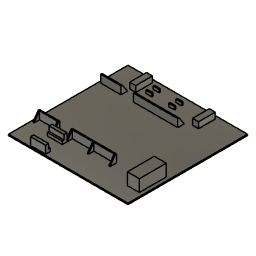
dysk v3 (Autodesk Fusion 360 design; units mm, degrees)
Autodesk Fusion 360 part; units mm, degrees
note: some values were not read from the file. Chosen so that the rebuilt part matches the saved one: which bodies a step acts on.
sketch "Szkic1" plane through (0, 0, 0) normal (0, 0, 1) x (1, 0, 0)
  line L0 (-100, 100) -> (100, 100)
  line L1 (100, 100) -> (100, -100)
  line L2 (100, -100) -> (-100, -100)
  line L3 (-100, -100) -> (-100, 100)
  dimension "d1" = 200
  dimension "d2" = 200
  constraint horizontal L0
  constraint vertical L1
  constraint horizontal L2
  constraint vertical L3
  measures "d1" distance of L0.start L0.end
  measures "d2" distance of L0.start L2.end
extrude "Wyciągnięcie proste1" add sketch "Szkic1" along normal blind 2 makes body 1
sketch "Szkic2" plane through (0, 0, 2) normal (0, 0, 1) x (-1, 0, 0)
  line L0 (100, 100) -> (-100, 100)
  line L1 (-100, 100) -> (-100, -100)
  line L2 (-100, -100) -> (100, -100)
  line L3 (100, -100) -> (100, 100)
  line L4 (95, 51) -> (65, 51)
  line L5 (95, 51) -> (65, 51)
  line L6 (65, 51) -> (65, 53)
  line L7 (65, 53) -> (95, 53)
  line L8 (95, 53) -> (95, 51)
  line L9 (95, -51) -> (65, -51)
  line L10 (65, -51) -> (65, -53)
  line L11 (65, -53) -> (95, -53)
  line L12 (95, -53) -> (95, -51)
  line L13 (40, -53) -> (-30, -53)
  line L14 (-30, -53) -> (-30, -51)
  line L15 (-30, -51) -> (40, -51)
  line L16 (40, -51) -> (40, -53)
  line L17 (40, 51) -> (-30, 51)
  line L18 (-30, 51) -> (-30, 53)
  line L19 (-30, 53) -> (40, 53)
  line L20 (40, 53) -> (40, 51)
  dimension "d10" = 30
  dimension "d11" = 5
  constraint horizontal L4
  constraint horizontal L5
  constraint vertical L6
  constraint horizontal L7
  constraint vertical L8
  constraint horizontal L9
  constraint vertical L10
  constraint horizontal L11
  constraint vertical L12
  constraint horizontal L13
  constraint vertical L14
  constraint horizontal L15
  constraint vertical L16
  constraint horizontal L17
  constraint vertical L18
  constraint horizontal L19
  constraint vertical L20
  measures "d10" distance of L10.end L11.end
  measures "d11" distance of L3 L12
extrude "Wyciągnięcie proste2" add sketch "Szkic2" along normal blind 13 separate body contours L4 L5 L6 L7 L8 | L9 L10 L11 L12 | L13 L14 L15 L16 | L17 L18 L19 L20 makes body 2 at (-16.6667, 53, 6.3333) makes body 3 at (-75, -53, 6.3333) makes body 4 at (-16.6667, -51, 6.3333) makes body 5 at (-75, 53, 6.3333)
sketch "Szkic3" plane through (-95, 0, 0) normal (-1, 0, 0) x (0, -1, 0)
  line L0 (51, 2) -> (53, 2)
  line L1 (53, 2) -> (53, 15)
  line L2 (53, 15) -> (51, 15)
  line L3 (51, 15) -> (51, 2)
  line L4 (53, 15) -> (62, 2)
  line L5 (62, 2) -> (51, 2)
  constraint coincident L1.end L2.start
  constraint coincident L0.start L3.end
extrude "Wyciągnięcie proste3" add sketch "Szkic3" along normal blind 2 separate body makes body 6
sketch "Szkic4" plane through (-95, 0, 0) normal (-1, 0, 0) x (0, -1, 0)
  line L0 (-53, 2) -> (-51, 2)
  line L1 (-51, 2) -> (-51, 15)
  line L2 (-51, 15) -> (-53, 15)
  line L3 (-53, 15) -> (-53, 2)
  line L4 (-53, 15) -> (-62, 2)
  line L5 (-62, 2) -> (-51, 2)
  constraint coincident L2.end L3.start
  constraint coincident L0.end L1.start
extrude "Wyciągnięcie proste4" add sketch "Szkic4" along normal blind 2 bodies 1 5
sketch "Szkic5" plane through (-65, 0, 0) normal (1, 0, 0) x (0, 1, 0)
  line L0 (51, 2) -> (53, 2)
  line L1 (53, 2) -> (53, 15)
  line L2 (53, 15) -> (51, 15)
  line L3 (51, 15) -> (51, 2)
  line L4 (53, 15) -> (62, 2)
  line L5 (62, 2) -> (51, 2)
  constraint coincident L1.end L2.start
  constraint coincident L0.start L3.end
extrude "Wyciągnięcie proste5" add sketch "Szkic5" along normal blind 2 bodies 1
sketch "Szkic6" plane through (-65, 0, 0) normal (1, 0, 0) x (0, 1, 0)
  line L0 (-53, 2) -> (-51, 2)
  line L1 (-51, 2) -> (-51, 15)
  line L2 (-51, 15) -> (-53, 15)
  line L3 (-53, 15) -> (-53, 2)
  line L4 (-53, 15) -> (-62, 2)
  line L5 (-62, 2) -> (-51, 2)
  constraint coincident L2.end L3.start
  constraint coincident L0.end L1.start
extrude "Wyciągnięcie proste6" add 1 faces at (30, -51.6667, 6.3333) along direction (1, 0, 0) blind 2 on bodies 4 bodies 1 2 3 6 4
extrude "Wyciągnięcie proste7" add sketch "Szkic6" along normal blind 2 bodies 1 6 3
sketch "Szkic7" plane through (-40, 0, 0) normal (-1, 0, 0) x (0, -1, 0)
  line L0 (51, 2) -> (53, 2)
  line L1 (53, 2) -> (53, 15)
  line L2 (53, 15) -> (51, 15)
  line L3 (51, 15) -> (51, 2)
  line L4 (53, 15) -> (62, 2)
  line L5 (62, 2) -> (51, 2)
  constraint coincident L1.end L2.start
  constraint coincident L0.start L3.end
extrude "Wyciągnięcie proste8" add sketch "Szkic7" along normal blind 2 bodies 1
sketch "Szkic8" plane through (32, 0, 0) normal (1, 0, 0) x (0, 1, 0)
  line L0 (-53, 2) -> (-51, 2)
  line L1 (-51, 2) -> (-51, 15)
  line L2 (-51, 15) -> (-53, 15)
  line L3 (-53, 15) -> (-53, 2)
  line L4 (-53, 15) -> (-62, 2)
  line L5 (-62, 2) -> (-51, 2)
  constraint coincident L2.end L3.start
  constraint coincident L0.end L1.start
extrude "Wyciągnięcie proste9" add sketch "Szkic8" along normal blind 2 bodies 1
sketch "Szkic9" plane through (30, 0, 0) normal (1, 0, 0) x (0, 1, 0)
  line L0 (51, 2) -> (53, 2)
  line L1 (53, 2) -> (53, 15)
  line L2 (53, 15) -> (51, 15)
  line L3 (51, 15) -> (51, 2)
  line L4 (53, 15) -> (62, 2)
  line L5 (62, 2) -> (51, 2)
  constraint coincident L1.end L2.start
  constraint coincident L0.start L3.end
extrude "Wyciągnięcie proste10" add sketch "Szkic9" along normal blind 2 bodies 1 2
sketch "Szkic10" plane through (-40, 0, 0) normal (-1, 0, 0) x (0, -1, 0)
  line L0 (-53, 2) -> (-51, 2)
  line L1 (-51, 2) -> (-51, 15)
  line L2 (-51, 15) -> (-53, 15)
  line L3 (-53, 15) -> (-53, 2)
  line L4 (-53, 15) -> (-62, 2)
  line L5 (-62, 2) -> (-51, 2)
  constraint coincident L2.end L3.start
  constraint coincident L0.end L1.start
extrude "Wyciągnięcie proste11" add sketch "Szkic10" along normal blind 2 bodies 1
sketch "Szkic11" plane through (0, 0, 2) normal (0, 0, 1) x (-1, 0, 0)
  line L0 (40, -62) -> (40, -53)
  line L1 (40, -53) -> (-30, -53)
  line L2 (-30, -53) -> (-30, -62)
  line L3 (-30, -62) -> (-32, -62)
  line L4 (-32, -62) -> (-32, -51)
  line L5 (-32, -51) -> (42, -51)
  line L6 (42, -51) -> (42, -62)
  line L7 (42, -62) -> (40, -62)
  line L8 (63, -51) -> (97, -51)
  line L9 (97, -51) -> (97, -62)
  line L10 (97, -62) -> (95, -62)
  line L11 (95, -62) -> (95, -53)
  line L12 (95, -53) -> (65, -53)
  line L13 (65, -53) -> (65, -62)
  line L14 (65, -62) -> (63, -62)
  line L15 (63, -62) -> (63, -51)
  line L16 (100, 100) -> (-100, 100)
  line L17 (-100, 100) -> (-100, -100)
  line L18 (-100, -100) -> (100, -100)
  line L19 (100, -100) -> (100, 100)
  line L20 (65, 62) -> (65, 53)
  line L21 (65, 53) -> (95, 53)
  line L22 (95, 53) -> (95, 51)
  line L23 (95, 51) -> (63, 51)
  line L24 (63, 51) -> (63, 62)
  line L25 (63, 62) -> (65, 62)
  line L26 (42, 51) -> (-34, 51)
  line L27 (-34, 51) -> (-34, 62)
  line L28 (-34, 62) -> (-32, 62)
  line L29 (-32, 62) -> (-32, 53)
  line L30 (-32, 53) -> (40, 53)
  line L31 (40, 53) -> (40, 62)
  line L32 (40, 62) -> (42, 62)
  line L33 (42, 62) -> (42, 51)
  line L34 (4, -53) -> (6, -53)
  line L35 (6, -53) -> (6, -62)
  line L36 (6, -62) -> (4, -62)
  line L37 (4, -62) -> (4, -53)
  dimension "d32" = 34
  dimension "d33" = 2
  constraint horizontal L34
  constraint vertical L35
  constraint horizontal L36
  constraint vertical L37
  constraint coincident L1 L34.start
  measures "d32" distance of L2 L37
  measures "d33" distance of L35.end L36.end
sketch "Szkic12" plane through (-6, 0, 0) normal (-1, 0, 0) x (0, -1, 0)
  line L0 (-62, 2) -> (-53, 2)
  line L1 (-53, 2) -> (-53, 15)
  line L2 (-53, 15) -> (-62, 15)
  line L3 (-62, 15) -> (-62, 2)
  line L4 (-53, 15) -> (-62, 2)
  line L5 (-53, 15) -> (-62, 2)
  line L6 (-51, 2) -> (-51, 15)
  line L7 (-51, 15) -> (-53, 15)
  constraint coincident L1.end L2.start
  constraint coincident L0.start L3.end
  constraint perpendicular L0 L6
  constraint perpendicular L1 L7
extrude "Wyciągnięcie proste13" add sketch "Szkic12" against normal blind 2 contours L0 L1 L4 L5 bodies 1
sketch "Szkic13" plane through (0, 0, 2) normal (0, 0, 1) x (-1, 0, 0)
  line L0 (4, -62) -> (4, -53)
  line L1 (4, -53) -> (-30, -53)
  line L2 (-30, -53) -> (-30, -62)
  line L3 (-30, -62) -> (-32, -62)
  line L4 (-32, -62) -> (-32, -51)
  line L5 (-32, -51) -> (42, -51)
  line L6 (42, -51) -> (42, -62)
  line L7 (42, -62) -> (40, -62)
  line L8 (40, -62) -> (40, -53)
  line L9 (40, -53) -> (6, -53)
  line L10 (6, -53) -> (6, -62)
  line L11 (6, -62) -> (4, -62)
  line L12 (63, -51) -> (97, -51)
  line L13 (97, -51) -> (97, -62)
  line L14 (97, -62) -> (95, -62)
  line L15 (95, -62) -> (95, -53)
  line L16 (95, -53) -> (65, -53)
  line L17 (65, -53) -> (65, -62)
  line L18 (65, -62) -> (63, -62)
  line L19 (63, -62) -> (63, -51)
  line L20 (100, 100) -> (-100, 100)
  line L21 (-100, 100) -> (-100, -100)
  line L22 (-100, -100) -> (100, -100)
  line L23 (100, -100) -> (100, 100)
  line L24 (65, 62) -> (65, 53)
  line L25 (65, 53) -> (95, 53)
  line L26 (95, 53) -> (95, 51)
  line L27 (95, 51) -> (63, 51)
  line L28 (63, 51) -> (63, 62)
  line L29 (63, 62) -> (65, 62)
  line L30 (42, 51) -> (-34, 51)
  line L31 (-34, 51) -> (-34, 62)
  line L32 (-34, 62) -> (-32, 62)
  line L33 (-32, 62) -> (-32, 53)
  line L34 (-32, 53) -> (40, 53)
  line L35 (40, 53) -> (40, 62)
  line L36 (40, 62) -> (42, 62)
  line L37 (42, 62) -> (42, 51)
  line L38 (6, 53) -> (2, 53)
  line L39 (2, 53) -> (2, 61)
  line L40 (2, 61) -> (6, 61)
  line L41 (6, 61) -> (6, 53)
  dimension "d38" = 34
  dimension "d39" = 34
  constraint horizontal L38
  constraint vertical L39
  constraint horizontal L40
  constraint vertical L41
  constraint coincident L34 L38.start
  measures "d38" distance of L35 L41
  measures "d39" distance of L33 L39
extrude "Wyciągnięcie proste14" add 1 faces at (34, -56, 6.3333) along direction (-1, 0, 0) blind 4 on bodies 1 bodies 1
extrude "Wyciągnięcie proste15" cut 1 faces at (34, -56, 6.3333) along direction (-1, 0, 0) blind 2 on bodies 1 bodies 1
sketch "Szkic14" plane through (0, 0, 2) normal (0, 0, 1) x (-1, 0, 0)
  line L0 (-30, 62) -> (-30, 53)
  line L1 (-30, 53) -> (40, 53)
  line L2 (40, 53) -> (40, 62)
  line L3 (40, 62) -> (42, 62)
  line L4 (42, 62) -> (42, 51)
  line L5 (42, 51) -> (-32, 51)
  line L6 (-32, 51) -> (-32, 62)
  line L7 (-32, 62) -> (-30, 62)
  line L8 (4, -62) -> (4, -53)
  line L9 (4, -53) -> (-30, -53)
  line L10 (-30, -53) -> (-30, -62)
  line L11 (-30, -62) -> (-32, -62)
  line L12 (-32, -62) -> (-32, -51)
  line L13 (-32, -51) -> (42, -51)
  line L14 (42, -51) -> (42, -62)
  line L15 (42, -62) -> (40, -62)
  line L16 (40, -62) -> (40, -53)
  line L17 (40, -53) -> (6, -53)
  line L18 (6, -53) -> (6, -62)
  line L19 (6, -62) -> (4, -62)
  line L20 (63, -51) -> (97, -51)
  line L21 (97, -51) -> (97, -62)
  line L22 (97, -62) -> (95, -62)
  line L23 (95, -62) -> (95, -53)
  line L24 (95, -53) -> (65, -53)
  line L25 (65, -53) -> (65, -62)
  line L26 (65, -62) -> (63, -62)
  line L27 (63, -62) -> (63, -51)
  line L28 (100, 100) -> (-100, 100)
  line L29 (-100, 100) -> (-100, -100)
  line L30 (-100, -100) -> (100, -100)
  line L31 (100, -100) -> (100, 100)
  line L32 (65, 62) -> (65, 53)
  line L33 (65, 53) -> (95, 53)
  line L34 (95, 53) -> (95, 51)
  line L35 (95, 51) -> (63, 51)
  line L36 (63, 51) -> (63, 62)
  line L37 (63, 62) -> (65, 62)
sketch "Szkic15" plane through (0, 0, 2) normal (0, 0, 1) x (-1, 0, 0)
  line L0 (6, 62) -> (4, 62)
  line L1 (4, 62) -> (4, 53)
  line L2 (4, 53) -> (6, 53)
  line L3 (6, 53) -> (6, 62)
  line L4 (-30, 53) -> (40, 53)
  line L5 (40, 53) -> (40, 62)
  dimension "d44" = 34
  dimension "d45" = 9
  constraint horizontal L0
  constraint vertical L1
  constraint horizontal L2
  constraint vertical L3
  constraint coincident L1.end L4
  measures "d44" distance of L3 L5
  measures "d45" distance of L0.start L2.end
sketch "Szkic16" plane through (-4, 0, 0) normal (1, 0, 0) x (0, 1, 0)
  line L0 (-62, 2) -> (-53, 2)
  line L1 (-53, 2) -> (-53, 15)
  line L2 (-53, 15) -> (-62, 15)
  line L3 (-62, 15) -> (-62, 2)
  line L4 (-53, 15) -> (-62, 2)
  line L5 (-51, 2) -> (-51, 15)
  line L6 (-51, 15) -> (-53, 15)
  constraint coincident L1.end L2.start
  constraint coincident L0.start L3.end
  constraint perpendicular L0 L5
  constraint perpendicular L1 L6
extrude "Wyciągnięcie proste17" add sketch "Szkic16" against normal blind 2 contours L0 L1 L4 bodies 1
sketch "Szkic17" plane through (0, 0, 2) normal (0, 0, 1) x (-1, 0, 0)
sketch "Sketch18" plane through (0, 0, 2) normal (0, 0, 1) x (-1, 0, 0)
split "Split1" by plane through (0, 0, 2) normal (0, 0, 1) bodies 1 makes body 7 at (7.3333, -51, 6.3333) makes body 8 at (-85.6667, 51, 10.6667) makes body 9 at (-84.3333, -51, 6.3333) makes body 10 at (-17.3333, 51, 6.3333)
combine "Combine1" operation add target body 6 tool bodies 9
move_body "Move1" bodies 6 7 to x (1, 0, 0) y (0, 1, 0) z (0, 0, 1) at (0, -0.2, 0)
move_body "Move2" bodies 8 10 to x (1, 0, 0) y (0, 1, 0) z (0, 0, 1) at (0, 0.2, 0)
sketch "Sketch19" plane through (0, 0, 2) normal (0, 0, 1) x (-1, 0, 0)
  line L0 (100, 100) -> (-100, 100)
  line L1 (-100, 100) -> (-100, -100)
  line L2 (-100, -100) -> (100, -100)
  line L3 (100, -100) -> (100, 100)
  line L4 (-3.9507, -74.0001) -> (6, -74.0001)
  line L5 (6, -74.0001) -> (6, -76)
  line L6 (6, -76) -> (-3.9507, -76)
  line L7 (-3.9507, -76) -> (-3.9507, -74.0001)
  line L8 (-4, -86) -> (6, -86)
  line L9 (6, -86) -> (6, -88)
  line L10 (6, -88) -> (-4, -88)
  line L11 (-4, -88) -> (-4, -86)
  line L12 (34, -73.992) -> (44.0493, -73.992)
  line L13 (44.0493, -73.992) -> (44.0493, -76)
  line L14 (44.0493, -76) -> (34, -76)
  line L15 (34, -76) -> (34, -73.992)
  line L16 (34, -86) -> (44, -86)
  line L17 (44, -86) -> (44, -88)
  line L18 (44, -88) -> (34, -88)
  line L19 (34, -88) -> (34, -86)
  line L20 (54, -67) -> (64, -67)
  line L21 (64, -67) -> (64, -95)
  line L22 (64, -95) -> (54, -95)
  line L23 (54, -95) -> (54, -67)
  line L24 (-28, -67) -> (-38, -67)
  line L25 (-38, -67) -> (-38, -95)
  line L26 (-38, -95) -> (-28, -95)
  line L27 (-28, -95) -> (-28, -67)
  dimension "d50" = 14
  dimension "d51" = 48
  dimension "d52" = 48
  dimension "d56" = 10
  dimension "d57" = 28
  constraint horizontal L4
  constraint vertical L5
  constraint horizontal L6
  constraint vertical L7
  constraint horizontal L8
  constraint vertical L9
  constraint horizontal L10
  constraint vertical L11
  constraint horizontal L12
  constraint vertical L13
  constraint horizontal L14
  constraint vertical L15
  constraint horizontal L16
  constraint vertical L17
  constraint horizontal L18
  constraint vertical L19
  constraint horizontal L20
  constraint vertical L21
  constraint horizontal L22
  constraint vertical L23
  constraint horizontal L24
  constraint vertical L25
  constraint horizontal L26
  constraint vertical L27
  measures "d50" distance of L4.start L10.end
  measures "d51" distance of L4.start L12.end
  measures "d52" distance of L10.end L17.end
  measures "d56" distance of L20.start L20.end
  measures "d57" distance of L20.start L22.end
extrude "Extrude18" add sketch "Sketch19" along normal blind 5 separate body contours L4 L5 L6 L7 | L8 L9 L10 L11 | L12 L13 L14 L15 | L16 L17 L18 L19 makes body 11 at (-37.3498, 73.992, 5.3333) makes body 12 at (-37.3333, 86, 3.6667) makes body 13 at (0.6338, 74.0001, 3.6667) makes body 14 at (0.6667, 86, 3.6667)
extrude "Extrude19" add sketch "Sketch19" along normal blind 10 separate body contours L20 L21 L22 L23 | L24 L25 L26 L27 makes body 15 at (34.6667, 76.3333, 2) makes body 16 at (-64, 76.3333, 5.3333)
sketch "Sketch20" plane through (0, 0, 2) normal (0, 0, 1) x (-1, 0, 0)
  line L0 (55, 75) -> (30, 75)
  line L1 (30, 75) -> (30, 83)
  line L2 (30, 83) -> (55, 83)
  line L3 (55, 83) -> (55, 75)
  line L4 (55, 80) -> (30, 80)
  line L5 (55, 89) -> (30, 89)
  line L6 (30, 89) -> (30, 97)
  line L7 (30, 97) -> (55, 97)
  line L8 (55, 97) -> (55, 89)
  line L9 (55, 92) -> (30, 92)
  constraint horizontal L0
  constraint vertical L1
  constraint horizontal L2
  constraint vertical L3
  constraint coincident L3 L4.start
  constraint coincident L1 L4.end
  constraint perpendicular L1 L4
  constraint horizontal L5
  constraint vertical L6
  constraint horizontal L7
  constraint vertical L8
  constraint coincident L8 L9.start
  constraint coincident L6 L9.end
  constraint perpendicular L6 L9
extrude "Extrude20" add sketch "Sketch20" along normal blind 13 separate body contours L0 L1 L3 L4 makes body 17
extrude "Extrude21" add sketch "Sketch20" along normal blind 5 separate body contours L1 L2 L3 L4 makes body 18
extrude "Extrude22" add sketch "Sketch20" along normal blind 5 separate body contours L5 L6 L8 L9 makes body 19
extrude "Extrude23" add sketch "Sketch20" along normal blind 13 separate body contours L6 L7 L8 L9 makes body 20
combine "Combine2" operation add target body 19 tool bodies 20
combine "Combine3" operation add target body 18 tool bodies 17
move_body "Move3" bodies 18 to x (1, 0, 0) y (0, 1, 0) z (0, 0, 1) at (-10, 10, 0)
move_body "Move4" bodies 19 to x (1, 0, 0) y (0, 1, 0) z (0, 0, 1) at (-10, 0, 0)
move_body "Move5" bodies 18 to x (1, 0, 0) y (0, 1, 0) z (0, 0, 1) at (0, 3, 0)
move_body "Move6" bodies 19 to x (1, 0, 0) y (0, 1, 0) z (0, 0, 1) at (0, -1, 0)
sketch "Sketch21" plane through (0, 0, 2) normal (0, 0, 1) x (-1, 0, 0)
  line L0 (-74, 80) -> (-94, 80)
  line L1 (-94, 80) -> (-94, 30)
  line L2 (-94, 30) -> (-74, 30)
  line L3 (-74, 30) -> (-74, 80)
  line L4 (-100, 100) -> (-100, -100)
  dimension "d68" = 50
  dimension "d69" = 20
  dimension "d70" = 6
  constraint horizontal L0
  constraint vertical L1
  constraint horizontal L2
  constraint vertical L3
  measures "d68" distance of L0.start L2.end
  measures "d69" distance of L0.start L0.end
  measures "d70" distance of L1 L4
move_body "Move7" bodies 15 to x (1, 0, 0) y (0, 1, 0) z (0, 0, 1) at (13, 0, 0)
extrude "Extrude24" add sketch "Sketch21" along normal blind 20 separate body makes body 21
move_body "Move8" bodies 21 to x (1, 0, 0) y (0, 1, 0) z (0, 0, 1) at (0, 5, 0)
extrude "Extrude25" cut 1 faces at (87.3333, -25, 8.6667) along direction (0, -1, 0) blind 5 on bodies 21 bodies 21
